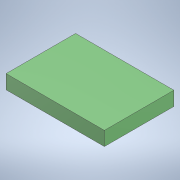
# Autodesk Inventor part: book
Saved by Autodesk Inventor 2022 (Build 260153000, 153)
## iProperties
Created: 2022-06-13
Part Number: book
Material: 一般
Document SubType Name: Modeling
Designer: yuto6
Density: 1 g/cm^3
Appearance: 既定
Author: yuto6
Autodesk Inventor part; units mm, degrees
ref_plane "YZ Plane" through (0, 0, 0) normal (1, 0, 0) x (0, 1, 0)
ref_plane "XZ Plane" through (0, 0, 0) normal (0, 1, 0) x (-1, 0, 0)
ref_plane "XY Plane" through (0, 0, 0) normal (0, 0, 1) x (1, 0, 0)
sketch "スケッチ1" plane through (0, 0, 0) normal (0, 1, 0) x (-1, 0, 0)
  line L0 (105, -148.5) -> (-105, -148.5)
  line L1 (-105, -148.5) -> (-105, 148.5)
  line L2 (-105, 148.5) -> (105, 148.5)
  line L3 (105, 148.5) -> (105, -148.5)
  line L4 (105, -148.5) -> (-105, 148.5) construction
  line L5 (-105, -148.5) -> (105, 148.5) construction
  point P0 (0, 0)
  dimension "d0" = 210
  dimension "d1" = 297
  constraints: 12 end point, 2 midpoint, 2 parallel, 1 horizontal, 1 perpendicular
  measures "d0" distance of L1.end L2.end
  measures "d1" distance of L2.end L0.start
extrude "押し出し1" add sketch "スケッチ1" along normal blind 60
mirror "ミラー1" about plane through (-105, 0, -148.5) normal (-1, 0, 0) of "押し出し1"
